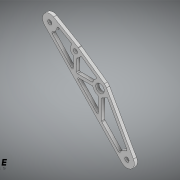
# Autodesk Inventor part: アームフレーム小
Saved by Autodesk Inventor 2020 (Build 240168000, 168)
## iProperties
Created: 2020-01-11
Part Number: アームフレーム小
Material: 一般
Document SubType Name: Modeling
Designer: tanjihayato
Density: 1 g/cm^3
Appearance: 既定
Author: tanjihayato
Autodesk Inventor part; units mm, degrees
ref_plane "YZ Plane" through (0, 0, 0) normal (1, 0, 0) x (0, 1, 0)
ref_plane "XZ Plane" through (0, 0, 0) normal (0, 1, 0) x (-1, 0, 0)
ref_plane "XY Plane" through (0, 0, 0) normal (0, 0, 1) x (1, 0, 0)
sketch "スケッチ1" plane through (0, 0, 0) normal (0, 0, 1) x (1, 0, 0)
  circle A0 centre (-1.9226, 44.1165) radius 4
  circle A1 centre (71.1898, -32.1215) radius 4
  circle A2 centre (71.1898, -32.1215) radius 2
  circle A3 centre (-1.9226, 44.1165) radius 2
  circle A4 centre (22.3463, 32.4678) radius 2
  circle A5 centre (45.6606, 13.5882) radius 4.025
  arc A6 (1.567, 50.1847) -> (-6.9748, 39.2714) centre (-1.9226, 44.1165) ccw
  arc A7 (66.1375, -36.9666) -> (77.3028, -28.7112) centre (71.1898, -32.1215) ccw
  arc A8 (51.7955, 17.0107) -> (49.703, 19.3336) centre (45.6606, 13.5882) ccw
  arc A9 (25.2234, 36.5571) -> (24.8388, 36.8022) centre (22.3463, 32.4678) ccw
  line L0 (1.567, 50.1847) -> (24.8388, 36.8022)
  line L1 (25.2234, 36.5571) -> (49.703, 19.3336)
  line L2 (51.7955, 17.0107) -> (77.3028, -28.7112)
  line L3 (-6.9748, 39.2714) -> (66.1375, -36.9666)
  point P0 (0, 0)
  point P1 (0, 0)
  dimension "d0" = 3
  dimension "d1" = 3
  dimension "d2" = 3
  dimension "d3" = 3
  constraints: 10 centre point, 8 end point, 8 point on circle, 8 tangent
  measures "d0" radial gap between concentric circles of A0 A6
  measures "d1" radial gap between concentric circles of A1 A7
  measures "d2" radial gap between concentric circles of A5 A8
  measures "d3" radial gap between concentric circles of A4 A9
extrude "押し出し1" add sketch "スケッチ1" along normal blind 3 contours A0 | A1 | L0 A9 L1 A8 L2 A7 L3 A6
extrude "押し出し2" cut sketch "スケッチ1" along normal blind 1 contours A0 | A1
sketch "スケッチ2" plane through (0, 0, 0) normal (0, 0, -1) x (-1, 0, 0)
  circle A0 centre (1.9226, 44.1165) radius 4 projected
  circle A1 centre (-71.1898, -32.1215) radius 4 projected
  arc A2 (-77.3028, -28.7112) -> (-66.1375, -36.9666) centre (-71.1898, -32.1215) ccw projected
  line L0 (6.9748, 39.2714) -> (-66.1375, -36.9666) projected
  arc A3 (6.9748, 39.2714) -> (-1.567, 50.1847) centre (1.9226, 44.1165) ccw projected
  line L1 (-24.8388, 36.8022) -> (-1.567, 50.1847) projected
  arc A4 (-24.8388, 36.8022) -> (-25.2234, 36.5571) centre (-22.3463, 32.4678) ccw projected
  line L2 (-49.703, 19.3336) -> (-25.2234, 36.5571) projected
  arc A5 (-49.703, 19.3336) -> (-51.7955, 17.0107) centre (-45.6606, 13.5882) ccw projected
  line L3 (-77.3028, -28.7112) -> (-51.7955, 17.0107) projected
  circle A6 centre (-22.3463, 32.4678) radius 2 projected
  circle A7 centre (-45.6606, 13.5882) radius 4.025 projected
  arc A8 (-23.3433, 34.2016) -> (-23.4971, 34.1035) centre (-22.3463, 32.4678) ccw
  line L4 (-23.3433, 34.2016) -> (-0.0714, 47.5841)
  arc A9 (4.8096, 41.3479) -> (-0.0714, 47.5841) centre (1.9226, 44.1165) ccw
  line L5 (4.8096, 41.3479) -> (-68.3028, -34.8902)
  arc A10 (-74.683, -30.1728) -> (-68.3028, -34.8902) centre (-71.1898, -32.1215) ccw
  line L6 (-74.683, -30.1728) -> (-49.1757, 15.5492)
  arc A11 (-47.9767, 16.8801) -> (-49.1757, 15.5492) centre (-45.6606, 13.5882) ccw
  line L7 (-47.9767, 16.8801) -> (-23.4971, 34.1035)
  circle A12 centre (1.9226, 44.1165) radius 7
  circle A13 centre (-71.1898, -32.1215) radius 7
  circle A14 centre (-45.6606, 13.5882) radius 7.025
  circle A15 centre (-22.3463, 32.4678) radius 5
  line L8 (-45.6606, 13.5882) -> (-5.0774, 13.5882) construction
  line L9 (-45.6606, 12.0882) -> (-5.0774, 12.0882)
  line L10 (-5.0774, 15.0882) -> (-45.6606, 15.0882)
  arc A16 (-45.6606, 15.0882) -> (-45.6606, 12.0882) centre (-45.6606, 13.5882) ccw
  arc A17 (-5.0774, 12.0882) -> (-5.0774, 15.0882) centre (-5.0774, 13.5882) ccw
  line L11 (-45.6606, 13.5882) -> (-45.6606, -36.9666) construction
  line L12 (-47.1606, 13.5882) -> (-47.1606, -36.9666)
  line L13 (-44.1606, -36.9666) -> (-44.1606, 13.5882)
  arc A18 (-44.1606, 13.5882) -> (-47.1606, 13.5882) centre (-45.6606, 13.5882) ccw
  arc A19 (-47.1606, -36.9666) -> (-44.1606, -36.9666) centre (-45.6606, -36.9666) ccw
  line L14 (-22.3463, 32.4678) -> (-21.0148, -7.0629) construction
  line L15 (-23.8454, 32.4173) -> (-22.514, -7.1134)
  line L16 (-19.5157, -7.0124) -> (-20.8471, 32.5183)
  arc A20 (-20.8471, 32.5183) -> (-23.8454, 32.4173) centre (-22.3463, 32.4678) ccw
  arc A21 (-22.514, -7.1134) -> (-19.5157, -7.0124) centre (-21.0148, -7.0629) ccw
  point P0 (0, 0)
  point P1 (-25.369, 13.5882)
  point P2 (-45.6606, -11.6892)
  point P3 (-38.7977, 15.0882)
  point P4 (-20.3735, 15.0882)
  point P5 (0.8334, 37.2018)
  point P6 (-5.0513, 44.7204)
  point P7 (-19.3707, 36.486)
  point P8 (-27.245, 31.4666)
  point P9 (-43.2679, 20.1931)
  point P10 (-44.1606, 6.7252)
  point P11 (-44.1606, -9.7159)
  point P12 (-23.2505, 12.0882)
  point P13 (-38.7977, 12.0882)
  point P14 (-47.1606, -12.8441)
  point P15 (-47.1606, 6.7252)
  point P16 (-51.9807, 10.5211)
  point P17 (-71.8842, -25.1561)
  point P18 (-64.3266, -30.744)
  point P19 (-21.6805, 12.7025)
  point P20 (-23.2618, 15.0882)
  point P21 (-23.6849, 27.6503)
  point P22 (-20.6866, 27.7513)
  point P23 (-20.2639, 15.2025)
  dimension "d8" = 3
  dimension "d9" = 3
  dimension "d10" = 3
  dimension "d11" = 3
  dimension "d12" = 3
  dimension "d13" = 3
  dimension "d14" = 3
  dimension "d17" = 3
  constraints: 32 end point, 20 point on circle, 14 centre point, 12 tangent, 3 midpoint, 3 parallel, 1 horizontal, 1 perpendicular, 7 other
  measures "d8" distance between parallel lines of L2 L7
  measures "d9" radial gap between concentric circles of A0 A12
  measures "d10" radial gap between concentric circles of A1 A13
  measures "d11" radial gap between concentric circles of A7 A14
  measures "d12" radial gap between concentric circles of A6 A15
  measures "d13" diameter of A17
  measures "d14" diameter of A19
  measures "d17" diameter of A21
extrude "押し出し3" cut sketch "スケッチ2" against normal through all contours A12 L5 L16 A15 L4 | L10 A14 L7 A15 L15 | L5 L13 A14 L9 | A14 L12 L5 A13 L6
fillet "フィレット1" radius 1 19 edges at (71.8842, -25.1561, 1.5) (64.3266, -30.744, 1.5) (47.1606, -12.8441, 1.5) (47.1606, 6.7252, 1.5) (51.9807, 10.5211, 1.5) (44.1606, 6.7252, 1.5) (44.1606, -9.7159, 1.5) (23.2505, 12.0882, 1.5) (23.2618, 15.0882, 1.5) (38.7977, 12.0882, 1.5) (38.7977, 15.0882, 1.5) (43.2679, 20.1931, 1.5) (23.6849, 27.6503, 1.5) (27.245, 31.4666, 1.5) (20.2639, 15.2025, 1.5) (20.6866, 27.7513, 1.5) (19.3707, 36.486, 1.5) (5.0513, 44.7204, 1.5) (-0.8334, 37.2018, 1.5)
sketch "スケッチ3" plane through (0, 0, 0) normal (0, 0, -1) x (-1, 0, 0)
  arc A0 (-64.8037, -29.2549) -> (-70.3207, -25.1757) centre (-71.1898, -32.1215) ccw projected
  arc A1 (-71.0698, -23.6962) -> (-70.3207, -25.1757) centre (-70.1965, -24.1834) ccw projected
  line L0 (-71.0698, -23.6962) -> (-52.797, 9.0579) projected
  arc A2 (-51.1432, 9.196) -> (-52.797, 9.0579) centre (-51.9237, 8.5707) ccw projected
  arc A3 (-51.1432, 9.196) -> (-47.8491, 6.9128) centre (-45.6606, 13.5882) ccw projected
  arc A4 (-47.1606, 5.9625) -> (-47.8491, 6.9128) centre (-48.1606, 5.9625) ccw projected
  line L1 (-47.1606, 5.9625) -> (-47.1606, -12.4421) projected
  arc A5 (-47.4389, -13.1343) -> (-47.1606, -12.4421) centre (-48.1606, -12.4421) ccw projected
  line L2 (-47.4389, -13.1343) -> (-63.1696, -29.5375) projected
  arc A6 (-64.8037, -29.2549) -> (-63.1696, -29.5375) centre (-63.8914, -28.8454) ccw projected
  line L3 (-24.296, 15.0882) -> (-38.035, 15.0882) projected
  arc A7 (-38.9852, 15.7767) -> (-38.035, 15.0882) centre (-38.035, 16.0882) ccw projected
  arc A8 (-38.9852, 15.7767) -> (-41.8628, 19.4981) centre (-45.6606, 13.5882) ccw projected
  arc A9 (-41.8976, 21.1572) -> (-41.8628, 19.4981) centre (-41.3222, 20.3394) ccw projected
  line L4 (-41.8976, 21.1572) -> (-28.3356, 30.6992) projected
  arc A10 (-26.8579, 30.3125) -> (-28.3356, 30.6992) centre (-27.7602, 29.8814) ccw projected
  arc A11 (-26.8579, 30.3125) -> (-24.2754, 27.855) centre (-22.3463, 32.4678) ccw projected
  arc A12 (-23.6618, 26.9661) -> (-24.2754, 27.855) centre (-24.6612, 26.9324) ccw projected
  line L5 (-23.6618, 26.9661) -> (-23.2966, 16.1219) projected
  arc A13 (-24.296, 15.0882) -> (-23.2966, 16.1219) centre (-24.296, 16.0882) ccw projected
  line L6 (-44.1606, -7.2284) -> (-44.1606, 5.9625) projected
  arc A14 (-43.4722, 6.9128) -> (-44.1606, 5.9625) centre (-43.1606, 5.9625) ccw projected
  arc A15 (-43.4722, 6.9128) -> (-38.9852, 11.3997) centre (-45.6606, 13.5882) ccw projected
  arc A16 (-38.035, 12.0882) -> (-38.9852, 11.3997) centre (-38.035, 11.0882) ccw projected
  line L7 (-38.035, 12.0882) -> (-25.595, 12.0882) projected
  arc A17 (-24.8733, 10.396) -> (-25.595, 12.0882) centre (-25.595, 11.0882) ccw projected
  line L8 (-24.8733, 10.396) -> (-42.4389, -7.9205) projected
  arc A18 (-44.1606, -7.2284) -> (-42.4389, -7.9205) centre (-43.1606, -7.2284) ccw projected
  line L9 (-18.2147, 37.1508) -> (-6.5004, 43.8871) projected
  arc A19 (-5.0114, 43.1572) -> (-6.5004, 43.8871) centre (-6.0019, 43.0202) ccw projected
  arc A20 (-5.0114, 43.1572) -> (-0.6744, 37.6161) centre (1.9226, 44.1165) ccw projected
  arc A21 (-0.3236, 35.9953) -> (-0.6744, 37.6161) centre (-1.0454, 36.6874) ccw projected
  line L10 (-0.3236, 35.9953) -> (-18.6225, 16.914) projected
  arc A22 (-20.3437, 17.5725) -> (-18.6225, 16.914) centre (-19.3443, 17.6062) ccw projected
  line L11 (-20.3437, 17.5725) -> (-20.6635, 27.067) projected
  arc A23 (-20.1111, 27.9952) -> (-20.6635, 27.067) centre (-19.6641, 27.1007) ccw projected
  arc A24 (-20.1111, 27.9952) -> (-18.4879, 35.6479) centre (-22.3463, 32.4678) ccw projected
  arc A25 (-18.2147, 37.1508) -> (-18.4879, 35.6479) centre (-17.7162, 36.2839) ccw projected
  circle A26 centre (1.9226, 44.1165) radius 4 projected
  circle A27 centre (-71.1898, -32.1215) radius 4 projected
  arc A28 (-77.3028, -28.7112) -> (-66.1375, -36.9666) centre (-71.1898, -32.1215) ccw projected
  line L12 (6.9748, 39.2714) -> (-66.1375, -36.9666) projected
  arc A29 (6.9748, 39.2714) -> (-1.567, 50.1847) centre (1.9226, 44.1165) ccw projected
  line L13 (-24.8388, 36.8022) -> (-1.567, 50.1847) projected
  arc A30 (-24.8388, 36.8022) -> (-25.2234, 36.5571) centre (-22.3463, 32.4678) ccw projected
  line L14 (-49.703, 19.3336) -> (-25.2234, 36.5571) projected
  arc A31 (-49.703, 19.3336) -> (-51.7955, 17.0107) centre (-45.6606, 13.5882) ccw projected
  line L15 (-77.3028, -28.7112) -> (-51.7955, 17.0107) projected
  circle A32 centre (-22.3463, 32.4678) radius 2 projected
  circle A33 centre (-45.6606, 13.5882) radius 4.025 projected
  circle A34 centre (1.9226, 44.1165) radius 2 projected
  circle A35 centre (-71.1898, -32.1215) radius 2 projected
  point P0 (0, 0)
